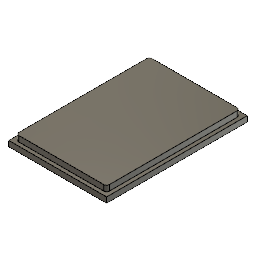
lid version 5 v1 (Autodesk Fusion 360 design; units mm, degrees)
Autodesk Fusion 360 part; units mm, degrees
sketch "Sketch1" plane through (0, 0, 0) normal (0, 1, 0) x (1, 0, 0) in component "Lid"
  line L0 (44.196, 63.5) -> (-44.196, 63.5)
  line L1 (-44.196, 63.5) -> (-44.196, -63.5)
  line L2 (-44.196, -63.5) -> (44.196, -63.5)
  line L3 (44.196, -63.5) -> (44.196, 63.5)
  line L4 (44.196, 63.5) -> (-44.196, -63.5) construction
  line L5 (-44.196, 63.5) -> (44.196, -63.5) construction
  dimension "d1" = 88.392
  dimension "d2" = 127
extrude "Extrude1" add sketch "Sketch1" along normal blind 5.08 in component "Lid"
sketch "Sketch3" plane through (0, 5.08, 0) normal (0, 1, 0) x (-1, 0, 0) in component "Lid"
  line L0 (-44.196, 63.5) -> (-44.196, -63.5)
  line L1 (-44.196, -63.5) -> (44.196, -63.5)
  line L2 (44.196, -63.5) -> (44.196, 63.5)
  line L3 (44.196, 63.5) -> (-44.196, 63.5)
  line L4 (-40.894, -60.198) -> (40.894, -60.198)
  line L5 (40.894, -60.198) -> (40.894, 60.198)
  line L6 (40.894, 60.198) -> (-40.894, 60.198)
  line L7 (-40.894, 60.198) -> (-40.894, -60.198)
  line L8 (-40.894, -60.198) -> (40.894, 60.198) construction
  line L9 (40.894, -60.198) -> (-40.894, 60.198) construction
  dimension "d6" = 81.788
  dimension "d7" = 120.396
extrude "Extrude2" add sketch "Sketch3" along normal blind 5.08 contours L4 L5 L6 L7 in component "Lid"
fillet "Fillet1" radius 2.54 4 edges at (-40.894, 7.62, -60.198) (40.894, 7.62, -60.198) (40.894, 7.62, 60.198) (-40.894, 7.62, 60.198) in component "Lid"
component "Lid" placed x (1, 0, 0) y (0, 1, 0) z (0, 0, 1) at (0, 0, 0)
